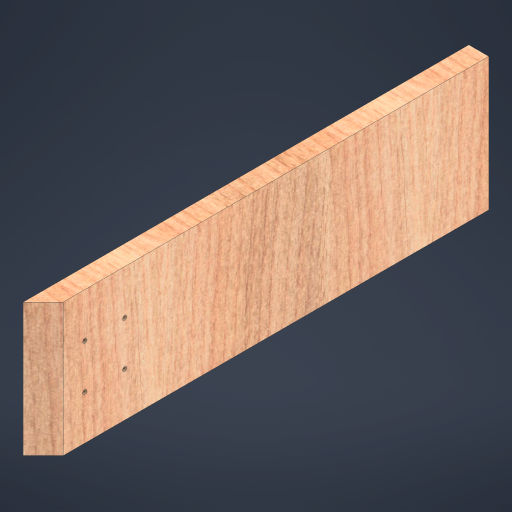
# Autodesk Inventor part: BUMP_002_Wood2
Saved by Autodesk Inventor 2024.2 (Build 282272000, 272)
## iProperties
Created: 2024-08-06
Part Number: BUMP_002_Wood2
Material: Wood (Birch)
Document SubType Name: Modeling
Designer: Bryan
Density: 0.55 g/cm^3
Appearance: Birch - Natural Polished
Author: Bryan
Autodesk Inventor part; units mm, degrees
ref_plane "YZ Plane" through (0, 0, 0) normal (1, 0, 0) x (0, 1, 0)
ref_plane "XZ Plane" through (0, 0, 0) normal (0, 1, 0) x (-1, 0, 0)
ref_plane "XY Plane" through (0, 0, 0) normal (0, 0, 1) x (1, 0, 0)
sketch "Sketch2" plane through (0, 0, 0) normal (0, 1, 0) x (-1, 0, 0)
  line L0 (0, 0) -> (0, -812.8)
  line L1 (19.05, 19.05) -> (19.05, -831.85)
  line L2 (19.05, -831.85) -> (0, -812.8)
  line L3 (19.05, 19.05) -> (0, 0)
  point P0 (19.05, -406.4)
  point P1 (0, -406.4)
  dimension "d2" = 812.8
  dimension "d3" = 850.9
  dimension "d4" = 19.05
  constraints: 8 end point, 2 midpoint, 2 vertical, 1 horizontal alignment
  measures "d2" distance of L0.start L0.end
  measures "d3" distance of L1.start L1.end
  measures "d4" distance between parallel lines of L0 L1
extrude "Extrusion1" add sketch "Sketch2" along normal blind 127
sketch "Sketch3" plane through (0, 0, 0) normal (1, 0, 0) x (0, 0, -1)
  line L0 (0, 0) -> (812.8, 0) construction
  line L1 (812.8, 0) -> (812.8, 127) construction
  line L2 (0, 127) -> (812.8, 127) construction
  line L3 (0, 0) -> (0, 127) construction
  line L4 (0, 84.6667) -> (20.574, 84.6667) construction
  circle A0 centre (20.574, 84.6667) radius 1.905
  circle A1 centre (58.674, 84.6667) radius 1.905
  circle A2 centre (96.774, 84.6667) radius 1.905 construction
  circle A3 centre (20.574, 42.3333) radius 1.905
  circle A4 centre (58.674, 42.3333) radius 1.905
  circle A5 centre (96.774, 42.3333) radius 1.905 construction
  line L5 (406.4, 127) -> (406.4, 0) construction
  circle A6 centre (792.226, 84.6667) radius 1.905
  circle A7 centre (754.126, 84.6667) radius 1.905
  circle A8 centre (716.026, 84.6667) radius 1.905 construction
  circle A9 centre (792.226, 42.3333) radius 1.905
  circle A10 centre (754.126, 42.3333) radius 1.905
  circle A11 centre (716.026, 42.3333) radius 1.905 construction
  point P0 (10.287, 84.6667)
  dimension "d7" = 20.574
  dimension "d8" = 42.3333
  dimension "d9" = 3.81
  dimension "d12" = 38.1
  dimension "d15" = 42.3333
  constraints: 12 centre point, 7 symmetric about line, 4 end point, 3 midpoint, 2 coincident, 2 horizontal, 1 point on line, 1 vertical, 16 other
  measures "d7" distance of L4.start L4.end
  measures "d8" distance from line of point (10.287, 84.667) L2
  measures "d9" diameter of A0
  measures "d12" distance of A0.centre A1.centre
  measures "d15" distance of A0.centre A3.centre
extrude "Extrusion2" cut sketch "Sketch3" against normal blind 127
sketch "Sketch4" plane through (0, 127, 0) normal (0, 1, 0) x (1, 0, 0)
  line L0 (-19.05, 831.85) -> (-19.05, -19.05) projected
  line L1 (-19.05, 406.4) -> (0, 406.4)
  line L2 (0, 0) -> (0, 812.8) projected
  line L3 (0, 0) -> (0, 812.8) projected
  line L4 (0, 812.8) -> (-19.05, 831.85) projected
  line L5 (-19.05, 831.85) -> (-19.05, -19.05) projected
  line L6 (-19.05, -19.05) -> (0, 0) projected
  constraints: 2 end point, 2 midpoint
extrude "Extrusion3" cut sketch "Sketch4" against normal blind 127 contours L4 L2 L1 L0
body "Solid1"
